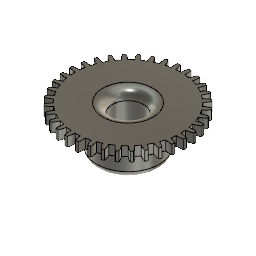
gear36 (Autodesk Fusion 360 design; units mm, degrees)
Autodesk Fusion 360 part; units mm, degrees
sketch "Sketch1" plane through (0, 0, 0) normal (0, 0, 1) x (1, 0, 0)
  circle A0 centre (0, 0) radius 5
  circle A1 centre (0, 0) radius 10
  dimension "d1" = 10
  dimension "d2" = 20
  constraint coincident A0.centre A1.centre
  measures "d1" diameter of A0
  measures "d2" diameter of A1
extrude "Extrude1" add sketch "Sketch1" along normal blind 11
sketch "Sketch2" plane through (0, 0, 11) normal (0, 0, 1) x (-1, 0, 0)
  circle A0 centre (0, 0) radius 5
  circle A1 centre (0, 0) radius 10
  circle A2 centre (0, 0) radius 19 construction
  circle A3 centre (0, 0) radius 18 construction
  circle A4 centre (0, 0) radius 16.83 construction
  line L0 (0, 0) -> (0, -19) construction
  line L1 (0, 0) -> (-1.571, -18.9349) construction
  line L2 (0, 0) -> (-0.785, -18.9838) construction
  arc A5 (-1.1772, -18.9635) -> (-0.3924, -18.9959) centre (0, 0) ccw
  arc A6 (-1.3916, -16.7724) -> (-1.1772, -18.9635) centre (4.7264, -17.28) ccw
  arc A7 (-0.3924, -18.9959) -> (0, -16.83) centre (-6.1737, -16.83) ccw
  line L3 (0, 0) -> (-3.142, -18.7384) construction
  arc A8 (-2.7832, -16.5983) -> (-1.3916, -16.7724) centre (0, 0) ccw
  arc A9 (1.5421, -16.7592) -> (2.1336, -18.8798) centre (7.6553, -16.1967) ccw
  arc A10 (2.9122, -18.7755) -> (2.9225, -16.5743) centre (-3.1574, -17.6464) ccw
  arc A11 (2.1336, -18.8798) -> (2.9122, -18.7755) centre (0, 0) ccw
  arc A12 (4.4288, -16.2368) -> (5.3796, -18.2225) centre (10.3515, -14.6213) ccw
  arc A13 (6.1282, -17.9846) -> (5.7562, -15.815) centre (-0.0452, -17.9265) ccw
  arc A14 (5.3796, -18.2225) -> (6.1282, -17.9846) centre (0, 0) ccw
  arc A15 (7.181, -15.2211) -> (8.4622, -17.0115) centre (12.7332, -12.6017) ccw
  arc A16 (9.1581, -16.6472) -> (8.415, -14.5752) centre (3.0684, -17.662) ccw
  arc A17 (8.4622, -17.0115) -> (9.1581, -16.6472) centre (0, 0) ccw
  arc A18 (9.7151, -13.7429) -> (11.2877, -15.2836) centre (14.728, -10.1991) ccw
  arc A19 (11.9098, -14.804) -> (10.8181, -12.8925) centre (6.0888, -16.8609) ccw
  arc A20 (11.2877, -15.2836) -> (11.9098, -14.804) centre (0, 0) ccw
  arc A21 (11.9539, -11.8471) -> (13.7702, -13.0913) centre (16.2753, -7.4867) ccw
  arc A22 (14.2995, -12.511) -> (12.8925, -10.8181) centre (8.9242, -15.5474) ccw
  arc A23 (13.7702, -13.0913) -> (14.2995, -12.511) centre (0, 0) ccw
  arc A24 (13.8295, -9.5913) -> (15.8342, -10.5013) centre (17.3281, -4.5468) ccw
  arc A25 (16.2548, -9.8378) -> (14.5752, -8.415) centre (11.4884, -13.7616) ccw
  arc A26 (15.8342, -10.5013) -> (16.2548, -9.8378) centre (0, 0) ccw
  arc A27 (15.2849, -7.0441) -> (17.4172, -7.5921) centre (17.8544, -1.4687) ccw
  arc A28 (17.7161, -6.8657) -> (15.815, -5.7562) centre (13.7035, -11.5576) ccw
  arc A29 (17.4172, -7.5921) -> (17.7161, -6.8657) centre (0, 0) ccw
  arc A30 (16.2759, -4.2829) -> (18.471, -4.4523) centre (17.8382, 1.654) ccw
  arc A31 (18.6392, -3.6851) -> (16.5743, -2.9225) centre (15.5023, -9.0024) ccw
  arc A32 (18.471, -4.4523) -> (18.6392, -3.6851) centre (0, 0) ccw
  arc A33 (16.7724, -1.3916) -> (18.9635, -1.1772) centre (17.28, 4.7264) ccw
  arc A34 (18.9959, -0.3924) -> (16.83, 0) centre (16.83, -6.1737) ccw
  arc A35 (18.9635, -1.1772) -> (18.9959, -0.3924) centre (0, 0) ccw
  arc A36 (16.7592, 1.5421) -> (18.8798, 2.1336) centre (16.1967, 7.6553) ccw
  arc A37 (18.7755, 2.9122) -> (16.5743, 2.9225) centre (17.6464, -3.1574) ccw
  arc A38 (18.8798, 2.1336) -> (18.7755, 2.9122) centre (0, 0) ccw
  arc A39 (16.2368, 4.4288) -> (18.2225, 5.3796) centre (14.6213, 10.3515) ccw
  arc A40 (17.9846, 6.1282) -> (15.815, 5.7562) centre (17.9265, -0.0452) ccw
  arc A41 (18.2225, 5.3796) -> (17.9846, 6.1282) centre (0, 0) ccw
  arc A42 (15.2211, 7.181) -> (17.0115, 8.4622) centre (12.6017, 12.7332) ccw
  arc A43 (16.6472, 9.1581) -> (14.5752, 8.415) centre (17.662, 3.0684) ccw
  arc A44 (17.0115, 8.4622) -> (16.6472, 9.1581) centre (0, 0) ccw
  arc A45 (13.7429, 9.7151) -> (15.2836, 11.2877) centre (10.1991, 14.728) ccw
  arc A46 (14.804, 11.9098) -> (12.8925, 10.8181) centre (16.8609, 6.0888) ccw
  arc A47 (15.2836, 11.2877) -> (14.804, 11.9098) centre (0, 0) ccw
  arc A48 (11.8471, 11.9539) -> (13.0913, 13.7702) centre (7.4867, 16.2753) ccw
  arc A49 (12.511, 14.2995) -> (10.8181, 12.8925) centre (15.5474, 8.9242) ccw
  arc A50 (13.0913, 13.7702) -> (12.511, 14.2995) centre (0, 0) ccw
  arc A51 (9.5913, 13.8295) -> (10.5013, 15.8342) centre (4.5468, 17.3281) ccw
  arc A52 (9.8378, 16.2548) -> (8.415, 14.5752) centre (13.7616, 11.4884) ccw
  arc A53 (10.5013, 15.8342) -> (9.8378, 16.2548) centre (0, 0) ccw
  arc A54 (7.0441, 15.2849) -> (7.5921, 17.4172) centre (1.4687, 17.8544) ccw
  arc A55 (6.8657, 17.7161) -> (5.7562, 15.815) centre (11.5576, 13.7035) ccw
  arc A56 (7.5921, 17.4172) -> (6.8657, 17.7161) centre (0, 0) ccw
  arc A57 (4.2829, 16.2759) -> (4.4523, 18.471) centre (-1.654, 17.8382) ccw
  arc A58 (3.6851, 18.6392) -> (2.9225, 16.5743) centre (9.0024, 15.5023) ccw
  arc A59 (4.4523, 18.471) -> (3.6851, 18.6392) centre (0, 0) ccw
  arc A60 (1.3916, 16.7724) -> (1.1772, 18.9635) centre (-4.7264, 17.28) ccw
  arc A61 (0.3924, 18.9959) -> (0, 16.83) centre (6.1737, 16.83) ccw
  arc A62 (1.1772, 18.9635) -> (0.3924, 18.9959) centre (0, 0) ccw
  arc A63 (-1.5421, 16.7592) -> (-2.1336, 18.8798) centre (-7.6553, 16.1967) ccw
  arc A64 (-2.9122, 18.7755) -> (-2.9225, 16.5743) centre (3.1574, 17.6464) ccw
  arc A65 (-2.1336, 18.8798) -> (-2.9122, 18.7755) centre (0, 0) ccw
  arc A66 (-4.4288, 16.2368) -> (-5.3796, 18.2225) centre (-10.3515, 14.6213) ccw
  arc A67 (-6.1282, 17.9846) -> (-5.7562, 15.815) centre (0.0452, 17.9265) ccw
  arc A68 (-5.3796, 18.2225) -> (-6.1282, 17.9846) centre (0, 0) ccw
  arc A69 (-7.181, 15.2211) -> (-8.4622, 17.0115) centre (-12.7332, 12.6017) ccw
  arc A70 (-9.1581, 16.6472) -> (-8.415, 14.5752) centre (-3.0684, 17.662) ccw
  arc A71 (-8.4622, 17.0115) -> (-9.1581, 16.6472) centre (0, 0) ccw
  arc A72 (-9.7151, 13.7429) -> (-11.2877, 15.2836) centre (-14.728, 10.1991) ccw
  arc A73 (-11.9098, 14.804) -> (-10.8181, 12.8925) centre (-6.0888, 16.8609) ccw
  arc A74 (-11.2877, 15.2836) -> (-11.9098, 14.804) centre (0, 0) ccw
  arc A75 (-11.9539, 11.8471) -> (-13.7702, 13.0913) centre (-16.2753, 7.4867) ccw
  arc A76 (-14.2995, 12.511) -> (-12.8925, 10.8181) centre (-8.9242, 15.5474) ccw
  arc A77 (-13.7702, 13.0913) -> (-14.2995, 12.511) centre (0, 0) ccw
  arc A78 (-13.8295, 9.5913) -> (-15.8342, 10.5013) centre (-17.3281, 4.5468) ccw
  arc A79 (-16.2548, 9.8378) -> (-14.5752, 8.415) centre (-11.4884, 13.7616) ccw
  arc A80 (-15.8342, 10.5013) -> (-16.2548, 9.8378) centre (0, 0) ccw
  arc A81 (-15.2849, 7.0441) -> (-17.4172, 7.5921) centre (-17.8544, 1.4687) ccw
  arc A82 (-17.7161, 6.8657) -> (-15.815, 5.7562) centre (-13.7035, 11.5576) ccw
  arc A83 (-17.4172, 7.5921) -> (-17.7161, 6.8657) centre (0, 0) ccw
  arc A84 (-16.2759, 4.2829) -> (-18.471, 4.4523) centre (-17.8382, -1.654) ccw
  arc A85 (-18.6392, 3.6851) -> (-16.5743, 2.9225) centre (-15.5023, 9.0024) ccw
  arc A86 (-18.471, 4.4523) -> (-18.6392, 3.6851) centre (0, 0) ccw
  arc A87 (-16.7724, 1.3916) -> (-18.9635, 1.1772) centre (-17.28, -4.7264) ccw
  arc A88 (-18.9959, 0.3924) -> (-16.83, 0) centre (-16.83, 6.1737) ccw
  arc A89 (-18.9635, 1.1772) -> (-18.9959, 0.3924) centre (0, 0) ccw
  arc A90 (-16.7592, -1.5421) -> (-18.8798, -2.1336) centre (-16.1967, -7.6553) ccw
  arc A91 (-18.7755, -2.9122) -> (-16.5743, -2.9225) centre (-17.6464, 3.1574) ccw
  arc A92 (-18.8798, -2.1336) -> (-18.7755, -2.9122) centre (0, 0) ccw
  arc A93 (-16.2368, -4.4288) -> (-18.2225, -5.3796) centre (-14.6213, -10.3515) ccw
  arc A94 (-17.9846, -6.1282) -> (-15.815, -5.7562) centre (-17.9265, 0.0452) ccw
  arc A95 (-18.2225, -5.3796) -> (-17.9846, -6.1282) centre (0, 0) ccw
  arc A96 (-15.2211, -7.181) -> (-17.0115, -8.4622) centre (-12.6017, -12.7332) ccw
  arc A97 (-16.6472, -9.1581) -> (-14.5752, -8.415) centre (-17.662, -3.0684) ccw
  arc A98 (-17.0115, -8.4622) -> (-16.6472, -9.1581) centre (0, 0) ccw
  arc A99 (-13.7429, -9.7151) -> (-15.2836, -11.2877) centre (-10.1991, -14.728) ccw
  arc A100 (-14.804, -11.9098) -> (-12.8925, -10.8181) centre (-16.8609, -6.0888) ccw
  arc A101 (-15.2836, -11.2877) -> (-14.804, -11.9098) centre (0, 0) ccw
  arc A102 (-11.8471, -11.9539) -> (-13.0913, -13.7702) centre (-7.4867, -16.2753) ccw
  arc A103 (-12.511, -14.2995) -> (-10.8181, -12.8925) centre (-15.5474, -8.9242) ccw
  arc A104 (-13.0913, -13.7702) -> (-12.511, -14.2995) centre (0, 0) ccw
  arc A105 (-9.5913, -13.8295) -> (-10.5013, -15.8342) centre (-4.5468, -17.3281) ccw
  arc A106 (-9.8378, -16.2548) -> (-8.415, -14.5752) centre (-13.7616, -11.4884) ccw
  arc A107 (-10.5013, -15.8342) -> (-9.8378, -16.2548) centre (0, 0) ccw
  arc A108 (-7.0441, -15.2849) -> (-7.5921, -17.4172) centre (-1.4687, -17.8544) ccw
  arc A109 (-6.8657, -17.7161) -> (-5.7562, -15.815) centre (-11.5576, -13.7035) ccw
  arc A110 (-7.5921, -17.4172) -> (-6.8657, -17.7161) centre (0, 0) ccw
  arc A111 (-4.2829, -16.2759) -> (-4.4523, -18.471) centre (1.654, -17.8382) ccw
  arc A112 (-3.6851, -18.6392) -> (-2.9225, -16.5743) centre (-9.0024, -15.5023) ccw
  arc A113 (-4.4523, -18.471) -> (-3.6851, -18.6392) centre (0, 0) ccw
  arc A114 (-2.9225, -16.5743) -> (-2.7832, -16.5983) centre (0, 0) ccw
  arc A115 (0.1414, -16.8294) -> (1.5421, -16.7592) centre (0, 0) ccw
  arc A116 (0, -16.83) -> (0.1414, -16.8294) centre (0, 0) ccw
  arc A117 (3.0616, -16.5492) -> (4.4288, -16.2368) centre (0, 0) ccw
  arc A118 (2.9225, -16.5743) -> (3.0616, -16.5492) centre (0, 0) ccw
  arc A119 (5.8889, -15.7661) -> (7.181, -15.2211) centre (0, 0) ccw
  arc A120 (5.7562, -15.815) -> (5.8889, -15.7661) centre (0, 0) ccw
  arc A121 (8.5372, -14.504) -> (9.7151, -13.7429) centre (0, 0) ccw
  arc A122 (8.415, -14.5752) -> (8.5372, -14.504) centre (0, 0) ccw
  arc A123 (10.926, -12.8012) -> (11.9539, -11.8471) centre (0, 0) ccw
  arc A124 (10.8181, -12.8925) -> (10.926, -12.8012) centre (0, 0) ccw
  arc A125 (12.983, -10.7094) -> (13.8295, -9.5913) centre (0, 0) ccw
  arc A126 (12.8925, -10.8181) -> (12.983, -10.7094) centre (0, 0) ccw
  arc A127 (14.6454, -8.2923) -> (15.2849, -7.0441) centre (0, 0) ccw
  arc A128 (14.5752, -8.415) -> (14.6454, -8.2923) centre (0, 0) ccw
  arc A129 (15.8628, -5.6231) -> (16.2759, -4.2829) centre (0, 0) ccw
  arc A130 (15.815, -5.7562) -> (15.8628, -5.6231) centre (0, 0) ccw
  arc A131 (16.5983, -2.7832) -> (16.7724, -1.3916) centre (0, 0) ccw
  arc A132 (16.5743, -2.9225) -> (16.5983, -2.7832) centre (0, 0) ccw
  arc A133 (16.8294, 0.1414) -> (16.7592, 1.5421) centre (0, 0) ccw
  arc A134 (16.83, 0) -> (16.8294, 0.1414) centre (0, 0) ccw
  arc A135 (16.5492, 3.0616) -> (16.2368, 4.4288) centre (0, 0) ccw
  arc A136 (16.5743, 2.9225) -> (16.5492, 3.0616) centre (0, 0) ccw
  arc A137 (15.7661, 5.8889) -> (15.2211, 7.181) centre (0, 0) ccw
  arc A138 (15.815, 5.7562) -> (15.7661, 5.8889) centre (0, 0) ccw
  arc A139 (14.504, 8.5372) -> (13.7429, 9.7151) centre (0, 0) ccw
  arc A140 (14.5752, 8.415) -> (14.504, 8.5372) centre (0, 0) ccw
  arc A141 (12.8012, 10.926) -> (11.8471, 11.9539) centre (0, 0) ccw
  arc A142 (12.8925, 10.8181) -> (12.8012, 10.926) centre (0, 0) ccw
  arc A143 (10.7094, 12.983) -> (9.5913, 13.8295) centre (0, 0) ccw
  arc A144 (10.8181, 12.8925) -> (10.7094, 12.983) centre (0, 0) ccw
  arc A145 (8.2923, 14.6454) -> (7.0441, 15.2849) centre (0, 0) ccw
  arc A146 (8.415, 14.5752) -> (8.2923, 14.6454) centre (0, 0) ccw
  arc A147 (5.6231, 15.8628) -> (4.2829, 16.2759) centre (0, 0) ccw
  arc A148 (5.7562, 15.815) -> (5.6231, 15.8628) centre (0, 0) ccw
  arc A149 (2.7832, 16.5983) -> (1.3916, 16.7724) centre (0, 0) ccw
  arc A150 (2.9225, 16.5743) -> (2.7832, 16.5983) centre (0, 0) ccw
  arc A151 (-0.1414, 16.8294) -> (-1.5421, 16.7592) centre (0, 0) ccw
  arc A152 (0, 16.83) -> (-0.1414, 16.8294) centre (0, 0) ccw
  arc A153 (-3.0616, 16.5492) -> (-4.4288, 16.2368) centre (0, 0) ccw
  arc A154 (-2.9225, 16.5743) -> (-3.0616, 16.5492) centre (0, 0) ccw
  arc A155 (-5.8889, 15.7661) -> (-7.181, 15.2211) centre (0, 0) ccw
  arc A156 (-5.7562, 15.815) -> (-5.8889, 15.7661) centre (0, 0) ccw
  arc A157 (-8.5372, 14.504) -> (-9.7151, 13.7429) centre (0, 0) ccw
  arc A158 (-8.415, 14.5752) -> (-8.5372, 14.504) centre (0, 0) ccw
  arc A159 (-10.926, 12.8012) -> (-11.9539, 11.8471) centre (0, 0) ccw
  arc A160 (-10.8181, 12.8925) -> (-10.926, 12.8012) centre (0, 0) ccw
  arc A161 (-12.983, 10.7094) -> (-13.8295, 9.5913) centre (0, 0) ccw
  arc A162 (-12.8925, 10.8181) -> (-12.983, 10.7094) centre (0, 0) ccw
  arc A163 (-14.6454, 8.2923) -> (-15.2849, 7.0441) centre (0, 0) ccw
  arc A164 (-14.5752, 8.415) -> (-14.6454, 8.2923) centre (0, 0) ccw
  arc A165 (-15.8628, 5.6231) -> (-16.2759, 4.2829) centre (0, 0) ccw
  arc A166 (-15.815, 5.7562) -> (-15.8628, 5.6231) centre (0, 0) ccw
  arc A167 (-16.5983, 2.7832) -> (-16.7724, 1.3916) centre (0, 0) ccw
  arc A168 (-16.5743, 2.9225) -> (-16.5983, 2.7832) centre (0, 0) ccw
  arc A169 (-16.8294, -0.1414) -> (-16.7592, -1.5421) centre (0, 0) ccw
  arc A170 (-16.83, 0) -> (-16.8294, -0.1414) centre (0, 0) ccw
  arc A171 (-16.5492, -3.0616) -> (-16.2368, -4.4288) centre (0, 0) ccw
  arc A172 (-16.5743, -2.9225) -> (-16.5492, -3.0616) centre (0, 0) ccw
  arc A173 (-15.7661, -5.8889) -> (-15.2211, -7.181) centre (0, 0) ccw
  arc A174 (-15.815, -5.7562) -> (-15.7661, -5.8889) centre (0, 0) ccw
  arc A175 (-14.504, -8.5372) -> (-13.7429, -9.7151) centre (0, 0) ccw
  arc A176 (-14.5752, -8.415) -> (-14.504, -8.5372) centre (0, 0) ccw
  arc A177 (-12.8012, -10.926) -> (-11.8471, -11.9539) centre (0, 0) ccw
  arc A178 (-12.8925, -10.8181) -> (-12.8012, -10.926) centre (0, 0) ccw
  arc A179 (-10.7094, -12.983) -> (-9.5913, -13.8295) centre (0, 0) ccw
  arc A180 (-10.8181, -12.8925) -> (-10.7094, -12.983) centre (0, 0) ccw
  arc A181 (-8.2923, -14.6454) -> (-7.0441, -15.2849) centre (0, 0) ccw
  arc A182 (-8.415, -14.5752) -> (-8.2923, -14.6454) centre (0, 0) ccw
  arc A183 (-5.6231, -15.8628) -> (-4.2829, -16.2759) centre (0, 0) ccw
  arc A184 (-5.7562, -15.815) -> (-5.6231, -15.8628) centre (0, 0) ccw
  dimension "d5" = 38
  dimension "d6" = 36
  dimension "d7" = 33.66
  dimension "d8" = 1.571
  dimension "d9" = 0.786
  dimension "d10" = 0.7855
  dimension "d11" = 1.571
  dimension "d13" = 360
  dimension "d15" = 360
  constraint coincident A0.centre A1.centre
  constraint coincident A2 L0.end
  constraint vertical L0
  constraint coincident A2 L1.end
  constraint coincident A2 L2.end
  constraint coincident A2 A5.end
  constraint coincident A2 A5.start
  constraint midpoint L2.end A5
  constraint tangent L1 A6
  constraint coincident A4 A6.start
  constraint coincident L1 A6.start
  constraint tangent L0 A7
  constraint coincident A4 A7.end
  constraint coincident L0 A7.end
  constraint coincident A2 L3.end
  constraint coincident A4 A8.start
  constraint coincident L3 A8.start
  constraint tangent A8 A114
  measures "d5" diameter of A2
  measures "d6" diameter of A3
  measures "d7" diameter of A4
  measures "d8" horizontal distance of L0.end L1.end
  measures "d9" horizontal distance of L1.end L2.end
  measures "d10" distance of A5.start A5.end
  measures "d11" horizontal distance of L1.end L3.end
extrude "Extrude2" add sketch "Sketch2" along normal blind 3 contours A1 | A5 A6 A7 A8 A9 A10 A11 A12 A13 A14 A15 A16 A17 A18 A19 A20 A21 A22 A23 A24 A25 A26 A27 A28 A29 A30 A31 A32 A33 A34 A35 A36 A37 A38 A39 A40 A41 A42 A43 A44 A45 A46 A47 A48 A49 A50 A51 A52 A53 A54 A55 A56 A57 A58 A59 A60 A61 A62 A63 A64 A65 A66 A67 A68 A69 A70 A71 A72 A73 A74 A75 A76 A77 A78 A79 A80 A81 A82 A83 A84 A85 A86 A87 A88 A89 A90 A91 A92 A93 A94 A95 A96 A97 A98 A99 A100 A101 A102 A103 A104 A105 A106 A107 A108 A109 A110 A111 A112 A113 A114 A115 A116 A117 A118 A119 A120 A121 A122 A123 A124 A125 A126 A127 A128 A129 A130 A131 A132 A133 A134 A135 A136 A137 A138 A139 A140 A141 A142 A143 A144 A145 A146 A147 A148 A149 A150 A151 A152 A153 A154 A155 A156 A157 A158 A159 A160 A161 A162 A163 A164 A165 A166 A167 A168 A169 A170 A171 A172 A173 A174 A175 A176 A177 A178 A179 A180 A181 A182 A183 A184
fillet "Fillet1" radius 3 1 edges at (4.6616, -1.8081, 14)
fillet "Fillet2" radius 2 2 edges at (-4.6616, 1.8081, 0) (-9.3233, -3.6162, 0)
